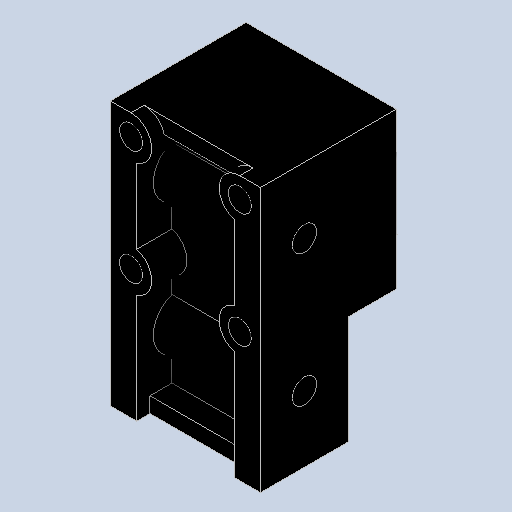
# Autodesk Inventor part: Y Axis Belt Stationary and Plate Spacer
Saved by Autodesk Inventor 2022 (Build 260153000, 153)
## iProperties
Created: 2021-10-13
Part Number: Y Axis Belt Stationary and Plate Spacer
Material: Generic
Document SubType Name: Modeling
Designer: Coy
Density: 1 g/cm^3
Appearance: Anodized - Black
Author: Coy
Autodesk Inventor part; units mm, degrees
ref_plane "YZ Plane" through (0, 0, 0) normal (1, 0, 0) x (0, 1, 0)
ref_plane "XZ Plane" through (0, 0, 0) normal (0, 1, 0) x (-1, 0, 0)
sketch "Sketch1" plane through (0, 0, 0) normal (1, 0, 0) x (0, 1, 0)
  line L0 (0, 0) -> (60, 0)
  line L1 (60, 0) -> (60, 20)
  line L2 (60, 20) -> (0, 20)
  line L3 (0, 20) -> (0, 0)
  line L4 (60, 10) -> (0, 10) construction
  line L5 (60, 10) -> (30, 10) construction
  line L6 (30, 10) -> (0, 10) construction
  circle A0 centre (45, 10) radius 2.75
  circle A1 centre (15, 10) radius 2.75
  dimension "d0" = 60
  dimension "d1" = 20
  dimension "d2" = 5.5
  dimension "d3" = 5.5
  constraints: 14 end point, 5 midpoint, 2 centre point, 2 parallel, 1 collinear, 1 horizontal, 1 perpendicular
  measures "d0" distance of L2.end L1.end
  measures "d1" distance of L1.end L0.end
  measures "d2" diameter of A0
  measures "d3" diameter of A1
extrude "Extrusion1" add sketch "Sketch1" against normal blind 6
sketch "Sketch2" plane through (-6, 0, 0) normal (-1, 0, 0) x (0, 0, 1)
  circle A0 centre (10, 45) radius 2.75 projected
  circle A1 centre (10, 15) radius 2.75 projected
  circle A2 centre (10, 45) radius 6.25
  circle A3 centre (10, 15) radius 6.25
  line L0 (20, 60) -> (0, 60) projected
  line L1 (12, 60) -> (12, 0)
  line L2 (8, 60) -> (8, 0)
  line L3 (0, 0) -> (20, 0) projected
  line L4 (0, 60) -> (0, 0) projected
  line L5 (20, 0) -> (20, 60) projected
  line L6 (12, 56.5) -> (17, 56.5)
  line L7 (17, 56.5) -> (17, 60)
  line L8 (8, 56.5) -> (3, 56.5)
  line L9 (3, 56.5) -> (3, 60)
  line L10 (8, 3.5) -> (3, 3.5)
  line L11 (3, 3.5) -> (3, 0)
  line L12 (12, 3.5) -> (17, 3.5)
  line L13 (17, 3.5) -> (17, 0)
  point P0 (12, 39.0786)
  point P1 (12, 50.9214)
  point P2 (8, 50.9214)
  point P3 (8, 39.0786)
  point P4 (8, 20.9214)
  point P5 (8, 9.0786)
  point P6 (12, 9.0786)
  point P7 (12, 20.9214)
  dimension "d6" = 3.5
  dimension "d7" = 8
  dimension "d8" = 8
  dimension "d9" = 3.5
  dimension "d10" = 3.5
  dimension "d11" = 3.5
  dimension "d16" = 3.5
  constraints: 20 end point, 15 point on line, 4 perpendicular, 2 centre point, 2 horizontal, 2 vertical, 1 coincident
  measures "d6" radial gap between concentric circles of A0 A2
  measures "d7" distance between parallel lines of L4 L2
  measures "d8" distance between parallel lines of L5 L1
  measures "d9" distance of L6.end L7.end
  measures "d10" distance of L8.end L9.end
  measures "d11" distance of L12.end L13.end
  measures "d16" radial gap between concentric circles of A1 A3
extrude "Extrusion2" add sketch "Sketch2" along normal blind 22.1 contours A0 L1 A2 | A0 L2 A2 L1 | L1 A2 L2 A0 | A0 L2 A2 | A2 L2 L0 L1 | L1 A3 L2 A2 | A2 L2 A3 L10 L11 L3 L4 L0 L9 L8 | L1 L0 L7 L6 | L1 A1 L2 A3 | A3 L1 A1 | L8 L9 L0 L2 | L2 A1 A3 | L2 A1 L1 A3 | A3 L1 L3 L2 | L2 L3 L11 L10 | L12 L13 L3 L1
sketch "Sketch3" plane through (-28.1, 0, 0) normal (-1, 0, 0) x (0, 0, 1)
  circle A0 centre (10, 45) radius 2.75 projected
  circle A1 centre (10, 15) radius 2.75 projected
  line L0 (20, 0) -> (20, 60) projected
  line L1 (17, 0) -> (20, 0) projected
  line L2 (0, 0) -> (17, 0) projected
  line L3 (0, 0) -> (20, 0) projected
  line L4 (0, 60) -> (0, 0) projected
  line L5 (20, 60) -> (17, 60) projected
  line L6 (17, 60) -> (0, 60) projected
  line L7 (20, 60) -> (17, 60) projected
  point P0 (3, 0)
  point P1 (3, 60)
extrude "Extrusion3" add sketch "Sketch3" along normal blind 6
sketch "Sketch4" plane through (0, 0, 0) normal (0, 0, -1) x (-1, 0, 0)
  line L0 (0, 42.25) -> (0, 47.75) projected
  line L1 (0, 0) -> (0, 60) projected
  line L2 (0, 50.3) -> (34.1, 50.3) construction
  line L3 (34.1, 60) -> (34.1, 0) projected
  line L4 (0, 34.3) -> (34.1, 34.3) construction
  line L5 (29.4, 55.3) -> (4.7, 55.3) construction
  line L6 (4.7, 55.3) -> (4.7, 29.3) construction
  line L7 (4.7, 29.3) -> (29.4, 29.3) construction
  line L8 (29.4, 29.3) -> (29.4, 55.3) construction
  circle A0 centre (29.4, 55.3) radius 2.6
  circle A1 centre (29.4, 29.3) radius 2.6
  circle A2 centre (4.7, 29.3) radius 2.6
  circle A3 centre (4.7, 55.3) radius 2.6
  line L9 (0, 60) -> (34.1, 60) projected
  line L10 (34.1, 24.6) -> (0, 24.6)
  line L11 (0, 60) -> (0, 0) projected
  dimension "d17" = 2.55
  dimension "d18" = 16
  dimension "d19" = 5.2
  dimension "d20" = 5.2
  dimension "d21" = 5.2
  dimension "d22" = 5.2
  dimension "d23" = 5
  dimension "d24" = 5
  dimension "d25" = 4.7
  dimension "d26" = 4.7
  dimension "d27" = 4.7
  dimension "d28" = 4.7
  constraints: 14 end point, 4 centre point, 4 coincident, 4 point on line, 3 parallel, 2 horizontal, 2 perpendicular
  measures "d17" distance from line of L2 L0.end
  measures "d18" distance between parallel lines of L2 L4
  measures "d19" diameter of A0
  measures "d20" diameter of A3
  measures "d21" diameter of A1
  measures "d22" diameter of A2
  measures "d23" distance between parallel lines of L2 L5
  measures "d24" distance between parallel lines of L7 L4
  measures "d25" distance from line of L9 L5.start
  measures "d26" distance between parallel lines of L8 L3
  measures "d27" distance between parallel lines of L0 L6
  measures "d28" distance between parallel lines of L7 L10
extrude "Extrusion4" add sketch "Sketch4" along normal blind 10.847
sketch "Sketch5" plane through (-4.7, 29.3, 0) normal (0, 0, -1) x (-1, 0, 0)
  line L0 (-4.7, 30.7) -> (-4.7, -4.7) projected
  line L1 (-4.7, -4.7) -> (29.4, -4.7) projected
  line L2 (29.4, -4.7) -> (29.4, 30.7) projected
  line L3 (29.4, 30.7) -> (-4.7, 30.7) projected
  circle A0 centre (24.7, 26) radius 2.6 projected
  circle A1 centre (24.7, 0) radius 2.6 projected
  circle A2 centre (0, 0) radius 2.6 projected
  circle A3 centre (0, 26) radius 2.6 projected
  point P0 (-4.7, -29.3)
extrude "Extrusion5" cut sketch "Sketch5" against normal through all contours A0 | A1 | A2 | A3
sketch "Sketch6" plane through (-34.1, 60, 20) normal (0, 0, 1) x (1, 0, 0)
  line L0 (34.1, 0) -> (34.1, -35.4) projected
  line L1 (34.1, -35.4) -> (0, -35.4) projected
  line L2 (0, -35.4) -> (0, 0) projected
  line L3 (0, 0) -> (34.1, 0) projected
  circle A0 centre (4.7, -4.7) radius 2.6 projected
  circle A1 centre (4.7, -30.7) radius 2.6 projected
  circle A2 centre (29.4, -30.7) radius 2.6 projected
  circle A3 centre (29.4, -4.7) radius 2.6 projected
  circle A4 centre (4.7, -4.7) radius 4.7
  circle A5 centre (29.4, -4.7) radius 4.7
  circle A6 centre (4.7, -30.7) radius 4.7
  circle A7 centre (29.4, -30.7) radius 4.7
  point P0 (34.1, -60)
  dimension "d33" = 2.1
  dimension "d34" = 2.1
  dimension "d35" = 2.1
  dimension "d36" = 2.1
  constraints: 4 centre point
  measures "d33" radial gap between concentric circles of A0 A4
  measures "d34" radial gap between concentric circles of A3 A5
  measures "d35" radial gap between concentric circles of A1 A6
  measures "d36" radial gap between concentric circles of A2 A7
extrude "Extrusion6" add sketch "Sketch6" against normal up to next contours A5 | A7 | A4 | A6
sketch "Sketch7" plane through (-34.1, 60, 20) normal (0, 0, 1) x (1, 0, 0)
  arc A0 (6, -9.2166) -> (6, -0.1834) centre (4.7, -4.7) ccw projected
  arc A1 (28.1, -0.1834) -> (28.1, -9.2166) centre (29.4, -4.7) ccw projected
  circle A2 centre (4.7, -4.7) radius 4.7
  circle A3 centre (29.4, -4.7) radius 4.7
  circle A4 centre (29.4, -30.7) radius 2.6 projected
  circle A5 centre (29.4, -4.7) radius 2.6 projected
  arc A6 (28.1, -0.1834) -> (28.1, -9.2166) centre (29.4, -4.7) ccw projected
  line L0 (28.1, -26.1834) -> (28.1, -9.2166) projected
  arc A7 (28.1, -26.1834) -> (28.1, -35.2166) centre (29.4, -30.7) ccw projected
  line L1 (28.1, -60) -> (28.1, -35.2166) projected
  line L2 (34.1, -60) -> (28.1, -60) projected
  line L3 (34.1, 0) -> (34.1, -60) projected
  line L4 (34.1, 0) -> (28.1, 0) projected
  line L5 (28.1, -0.1834) -> (28.1, 0) projected
  circle A8 centre (4.7, -30.7) radius 2.6 projected
  circle A9 centre (4.7, -4.7) radius 2.6 projected
  line L6 (6, 0) -> (0, 0) projected
  line L7 (0, -60) -> (0, 0) projected
  line L8 (6, -60) -> (0, -60) projected
  line L9 (6, -60) -> (6, -35.2166) projected
  arc A10 (6, -35.2166) -> (6, -26.1834) centre (4.7, -30.7) ccw projected
  line L10 (6, -26.1834) -> (6, -9.2166) projected
  arc A11 (6, -9.2166) -> (6, -0.1834) centre (4.7, -4.7) ccw projected
  line L11 (6, -0.1834) -> (6, 0) projected
  point P0 (29.4, 0)
  point P1 (4.7, 0)
  constraints: 2 coincident, 6 other
extrude "Extrusion7" cut sketch "Sketch7" against normal up to surface (3 mm away) contours A2 L6 L11 | L5 L4 A3
ref_plane "Work Plane2" through (0, 50.3, 20) normal (0, 1, 0) x (1, 0, 0)
sketch "Sketch9" plane through (0, 50.3, 20) normal (0, 1, 0) x (1, 0, 0)
  line L0 (-34.1, 30.847) -> (0, 30.847) projected
  line L1 (0, 33.247) -> (-34.1, 33.247)
  arc A0 (-0.8878, 31.7995) -> (0, 30.847) centre (0, 31.737) ccw
  line L2 (-3, 33.247) -> (-3, 30.847) construction
  line L3 (-7.3, 30.847) -> (-2.1, 30.847) projected
  line L4 (0, 30.847) -> (-34.1, 30.847) construction
  line L5 (0, 33.247) -> (0, 30.847)
  arc A1 (-3, 30.847) -> (-2.1122, 31.7995) centre (-3, 31.737) ccw
  line L6 (-34.1, 32.067) -> (-3, 32.067) construction
  line L7 (-1.8628, 32.067) -> (-1.1372, 32.067)
  arc A2 (-1.8628, 32.067) -> (-2.1122, 31.7995) centre (-1.8628, 31.817) ccw
  arc A3 (-0.8878, 31.7995) -> (-1.1372, 32.067) centre (-1.1372, 31.817) ccw
  arc A4 (-6, 30.847) -> (-5.1122, 31.7995) centre (-6, 31.737) ccw
  line L8 (-6, 33.247) -> (-6, 30.847) construction
  arc A5 (-3.8878, 31.7995) -> (-3, 30.847) centre (-3, 31.737) ccw
  line L9 (-4.1372, 32.067) -> (-4.8628, 32.067)
  arc A6 (-3.8878, 31.7995) -> (-4.1372, 32.067) centre (-4.1372, 31.817) ccw
  arc A7 (-4.8628, 32.067) -> (-5.1122, 31.7995) centre (-4.8628, 31.817) ccw
  line L10 (-9, 33.247) -> (-9, 30.847) construction
  arc A8 (-9, 30.847) -> (-8.1122, 31.7995) centre (-9, 31.737) ccw
  arc A9 (-7.8628, 32.067) -> (-8.1122, 31.7995) centre (-7.8628, 31.817) ccw
  line L11 (-7.1372, 32.067) -> (-7.8628, 32.067)
  arc A10 (-6.8878, 31.7995) -> (-7.1372, 32.067) centre (-7.1372, 31.817) ccw
  arc A11 (-6.8878, 31.7995) -> (-6, 30.847) centre (-6, 31.737) ccw
  line L12 (-12, 33.247) -> (-12, 30.847) construction
  arc A12 (-12, 30.847) -> (-11.1122, 31.7995) centre (-12, 31.737) ccw
  arc A13 (-10.8628, 32.067) -> (-11.1122, 31.7995) centre (-10.8628, 31.817) ccw
  line L13 (-10.1372, 32.067) -> (-10.8628, 32.067)
  arc A14 (-9.8878, 31.7995) -> (-10.1372, 32.067) centre (-10.1372, 31.817) ccw
  arc A15 (-9.8878, 31.7995) -> (-9, 30.847) centre (-9, 31.737) ccw
  line L14 (-15, 33.247) -> (-15, 30.847) construction
  arc A16 (-15, 30.847) -> (-14.1122, 31.7995) centre (-15, 31.737) ccw
  arc A17 (-13.8628, 32.067) -> (-14.1122, 31.7995) centre (-13.8628, 31.817) ccw
  line L15 (-13.1372, 32.067) -> (-13.8628, 32.067)
  arc A18 (-12.8878, 31.7995) -> (-13.1372, 32.067) centre (-13.1372, 31.817) ccw
  arc A19 (-12.8878, 31.7995) -> (-12, 30.847) centre (-12, 31.737) ccw
  line L16 (-18, 33.247) -> (-18, 30.847) construction
  arc A20 (-18, 30.847) -> (-17.1122, 31.7995) centre (-18, 31.737) ccw
  arc A21 (-16.8628, 32.067) -> (-17.1122, 31.7995) centre (-16.8628, 31.817) ccw
  line L17 (-16.1372, 32.067) -> (-16.8628, 32.067)
  arc A22 (-15.8878, 31.7995) -> (-16.1372, 32.067) centre (-16.1372, 31.817) ccw
  arc A23 (-15.8878, 31.7995) -> (-15, 30.847) centre (-15, 31.737) ccw
  line L18 (-21, 33.247) -> (-21, 30.847) construction
  arc A24 (-21, 30.847) -> (-20.1122, 31.7995) centre (-21, 31.737) ccw
  arc A25 (-19.8628, 32.067) -> (-20.1122, 31.7995) centre (-19.8628, 31.817) ccw
  line L19 (-19.1372, 32.067) -> (-19.8628, 32.067)
  arc A26 (-18.8878, 31.7995) -> (-19.1372, 32.067) centre (-19.1372, 31.817) ccw
  arc A27 (-18.8878, 31.7995) -> (-18, 30.847) centre (-18, 31.737) ccw
  line L20 (-24, 33.247) -> (-24, 30.847) construction
  arc A28 (-24, 30.847) -> (-23.1122, 31.7995) centre (-24, 31.737) ccw
  arc A29 (-22.8628, 32.067) -> (-23.1122, 31.7995) centre (-22.8628, 31.817) ccw
  line L21 (-22.1372, 32.067) -> (-22.8628, 32.067)
  arc A30 (-21.8878, 31.7995) -> (-22.1372, 32.067) centre (-22.1372, 31.817) ccw
  arc A31 (-21.8878, 31.7995) -> (-21, 30.847) centre (-21, 31.737) ccw
  line L22 (-27, 33.247) -> (-27, 30.847) construction
  arc A32 (-27, 30.847) -> (-26.1122, 31.7995) centre (-27, 31.737) ccw
  arc A33 (-25.8628, 32.067) -> (-26.1122, 31.7995) centre (-25.8628, 31.817) ccw
  line L23 (-25.1372, 32.067) -> (-25.8628, 32.067)
  arc A34 (-24.8878, 31.7995) -> (-25.1372, 32.067) centre (-25.1372, 31.817) ccw
  arc A35 (-24.8878, 31.7995) -> (-24, 30.847) centre (-24, 31.737) ccw
  line L24 (-30, 33.247) -> (-30, 30.847) construction
  arc A36 (-30, 30.847) -> (-29.1122, 31.7995) centre (-30, 31.737) ccw
  arc A37 (-28.8628, 32.067) -> (-29.1122, 31.7995) centre (-28.8628, 31.817) ccw
  line L25 (-28.1372, 32.067) -> (-28.8628, 32.067)
  arc A38 (-27.8878, 31.7995) -> (-28.1372, 32.067) centre (-28.1372, 31.817) ccw
  arc A39 (-27.8878, 31.7995) -> (-27, 30.847) centre (-27, 31.737) ccw
  line L26 (-33, 33.247) -> (-33, 30.847) construction
  arc A40 (-33, 30.847) -> (-32.1122, 31.7995) centre (-33, 31.737) ccw
  arc A41 (-31.8628, 32.067) -> (-32.1122, 31.7995) centre (-31.8628, 31.817) ccw
  line L27 (-31.1372, 32.067) -> (-31.8628, 32.067)
  arc A42 (-30.8878, 31.7995) -> (-31.1372, 32.067) centre (-31.1372, 31.817) ccw
  arc A43 (-30.8878, 31.7995) -> (-30, 30.847) centre (-30, 31.737) ccw
  line L28 (-36, 33.247) -> (-36, 30.847) construction
  arc A44 (-36, 30.847) -> (-35.1122, 31.7995) centre (-36, 31.737) ccw
  arc A45 (-34.8628, 32.067) -> (-35.1122, 31.7995) centre (-34.8628, 31.817) ccw
  line L29 (-34.1372, 32.067) -> (-34.8628, 32.067)
  arc A46 (-33.8878, 31.7995) -> (-34.1372, 32.067) centre (-34.1372, 31.817) ccw
  arc A47 (-33.8878, 31.7995) -> (-33, 30.847) centre (-33, 31.737) ccw
  line L30 (-34.1, 20) -> (-34.1, 30.847) projected
  line L31 (-34.1, 30.847) -> (-34.1, 33.247)
  point P0 (0, 20)
  point P1 (-0.8266, 32.067)
  point P2 (-2.1734, 32.067)
  point P3 (-34.1, 32.0642)
  dimension "d58" = 2.4
  dimension "d60" = 1.78
  dimension "d61" = 3
  dimension "d62" = 1.78
  dimension "d63" = 0.25
  dimension "d64" = 0.25
  dimension "d67" = 3
  constraints: 98 point on circle, 56 end point, 48 centre point, 9 symmetric about line, 5 point on line, 4 horizontal, 4 tangent, 1 collinear, 1 perpendicular, 1 vertical, 178 other
  measures "d60" diameter of A0
  measures "d61" distance between parallel lines of L5 L2
  measures "d62" diameter of A1
  measures "d63" radius of A2
  measures "d64" radius of A3
  measures "d67" distance of L8.start L10.start
extrude "Extrusion9" add sketch "Sketch9" against normal blind 16 contours L31 A46 A47 L0 | A40 A41 L27 A42 A43 L0 | A36 A37 L25 A38 A39 L0 | A32 A33 L23 A34 A35 L0 | A28 A29 L21 A30 A31 L0 | L0 A1 A2 L7 A3 A0 | A24 A25 L19 A26 A27 L0 | A20 A21 L17 A22 A23 L0 | L0 A4 A7 L9 A6 A5 | A16 A17 L15 A18 A19 L0 | L0 A8 A9 L11 A10 A11 | A12 A13 L13 A14 A15 L0
equation "\"d3\" = d2"
equation "\"d16\" = d6"
equation "\"d20\" = d19"
equation "\"d21\" = d19"
equation "\"d22\" = d19"
equation "\"d26\" = d25"
equation "\"d27\" = d25"
equation "\"d28\" = d25"
equation "\"d62\" = d60"
body "Solid1"
